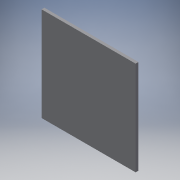
# Autodesk Inventor part: 바닥판
Saved by Autodesk Inventor 2017 (Build 210142000, 142)
## iProperties
Part Number: 바닥판
Material: 일반
Document SubType Name: Modeling
Designer: minom
Density: 1 g/cm^3
Appearance: 기본값
Author: minom
Autodesk Inventor part; units mm, degrees
ref_plane "YZ Plane" through (0, 0, 0) normal (1, 0, 0) x (0, 1, 0)
ref_plane "XZ Plane" through (0, 0, 0) normal (0, 1, 0) x (-1, 0, 0)
ref_plane "XY Plane" through (0, 0, 0) normal (0, 0, 1) x (1, 0, 0)
sketch "스케치1" plane through (0, 0, 0) normal (0, 1, 0) x (-1, 0, 0)
  line L0 (0, 0) -> (-330, 0)
  line L1 (-330, 0) -> (-330, -330)
  line L2 (-330, -330) -> (0, -330)
  line L3 (0, -330) -> (0, 0)
  dimension "d0" = 330
  dimension "d1" = 330
  constraints: 8 end point, 2 parallel, 1 horizontal, 1 perpendicular
  measures "d0" distance of L2.end L1.end
  measures "d1" distance of L1.end L0.end
extrude "돌출1" add sketch "스케치1" along normal blind 10
